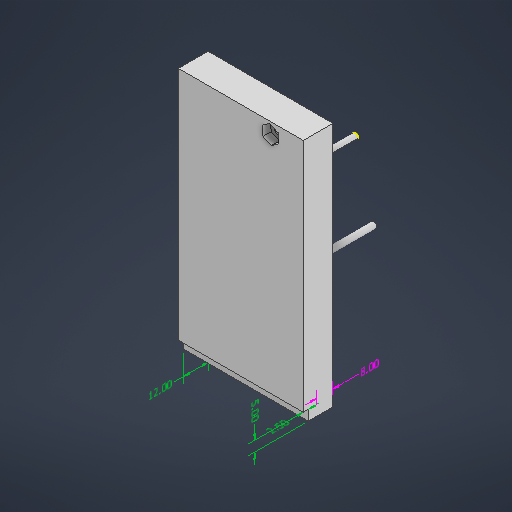
# Autodesk Inventor part: Cover of DC Housing
Saved by Autodesk Inventor 2026.2 (Build 302298010, 298A)
## iProperties
Created: 2026-04-19
Part Number: Cover of DC Housing
Material: Generic
Document SubType Name: Modeling
Designer: lenovo
Density: 1 g/cm^3
Appearance: Default
Author: lenovo
## iProperties of the stored document Cover of DC Housing_3DPrint.ipt
Created: 2026-04-19
Part Number: Cover of DC Housing_3DPrint
Material: Generic
Document SubType Name: Modeling
Designer: lenovo
Density: 1 g/cm^3
Appearance: Default
Author: lenovo
Autodesk Inventor part; units mm, degrees
ref_plane "YZ Plane" through (0, 0, 0) normal (1, 0, 0) x (0, 1, 0)
ref_plane "XZ Plane" through (0, 0, 0) normal (0, 1, 0) x (-1, 0, 0)
ref_plane "XY Plane" through (0, 0, 0) normal (0, 0, 1) x (1, 0, 0)
sketch "Sketch1" plane through (0, 0, 0) normal (0, 0, 1) x (1, 0, 0)
  line L0 (0, 0) -> (0, 120)
  line L1 (0, 120) -> (61, 120)
  line L2 (61, 120) -> (61, 0)
  line L3 (61, 0) -> (0, 0)
  line L4 (0, 5) -> (61, 5)
  line L5 (0, 110) -> (61, 110)
  dimension "d0" = 120
  dimension "d1" = 61
  dimension "d14" = 10
  dimension "d15" = 5
  constraints: 12 end point, 4 perpendicular, 4 point on line, 1 horizontal, 1 vertical
  measures "d0" distance of L0.start L0.end
  measures "d1" distance of L0.end L1.end
  measures "d14" distance between parallel lines of L5 L1
  measures "d15" distance between parallel lines of L3 L4
extrude "Extrusion1" add sketch "Sketch1" along normal blind 14.5 contours L0 L5 L2 L4 | L0 L1 L2 L5
extrude "Extrusion2" cut sketch "Sketch1" along normal blind 11.5 contours L0 L5 L2 L4
extrude "Extrusion3" add sketch "Sketch1" along normal blind 12 contours L0 L4 L2 L3
sketch "Sketch2" plane through (61, 5, 14.5) normal (1, 0, 0) x (0, 0, -1)
  line L0 (14.5, 115) -> (0, 115) projected
  line L1 (14.5, 115) -> (0, 115)
  line L2 (0, 0) -> (0, 115) projected
  line L3 (0, 115) -> (0, 0)
  line L4 (0, 0) -> (14.5, 0)
  line L5 (14.5, 0) -> (14.5, 115)
  point P0 (14.5, -5)
  constraints: 8 end point, 2 collinear, 2 perpendicular
extrude "Extrusion4" add sketch "Sketch2" against normal blind 1.5
sketch "Sketch3" plane through (0, 5, 14.5) normal (-1, 0, 0) x (0, 0, 1)
  line L0 (-14.5, 115) -> (-14.5, 105) projected
  line L1 (-14.5, 115) -> (0, 115) projected
  line L2 (-14.5, 115) -> (0, 115)
  line L3 (0, 0) -> (0, 115) projected
  line L4 (0, 115) -> (0, 0)
  line L5 (0, 0) -> (-14.5, 0)
  line L6 (-14.5, 0) -> (-14.5, 115)
  point P0 (-14.5, -5)
  constraints: 8 end point, 3 perpendicular, 1 horizontal
extrude "Extrusion5" add sketch "Sketch3" against normal blind 1.5
sketch "Sketch4" plane through (0, 0, 14.5) normal (0, 0, 1) x (1, 0, 0)
  circle A0 centre (45, 114.5) radius 2.25
  line L0 (61, 120) -> (0, 120) projected
  line L1 (45, 116.75) -> (46.9486, 115.625)
  line L2 (46.9486, 115.625) -> (46.9486, 113.375)
  line L3 (46.9486, 113.375) -> (45, 112.25)
  line L4 (45, 112.25) -> (43.0514, 113.375)
  line L5 (43.0514, 113.375) -> (43.0514, 115.625)
  line L6 (43.0514, 115.625) -> (45, 116.75)
  line L7 (0, 120) -> (0, 5) projected
  point P0 (0, 0)
  point P1 (30.5, 120)
  dimension "d23" = 4.5
  dimension "d60" = 45
  constraints: 12 end point, 1 coincident, 1 midpoint, 1 vertical alignment, 15 other
  measures "d60" distance from line of L7 point (45, 114.5)
hole "Hole1" at (45, 114.5, 14.5) direction (0, 0, -1) diameter 4.5 end through all counterbore diameter 9 counterbore depth 4
sketch "Sketch8" plane through (0, 0, 11.5) normal (0, 0, -1) x (-1, 0, 0)
  line L0 (-59.5, 110) -> (-1.5, 110) projected
  line L1 (-45, 110) -> (-45, 93)
  circle A0 centre (-45, 93) radius 1.4
  line L2 (-46.4, 93) -> (-43.6, 93)
  circle A1 centre (-36, 60) radius 1.4
  circle A2 centre (-54, 60) radius 1.4
  line L3 (-61, 0) -> (-61, 120) projected
  line L4 (-59.5, 110) -> (-59.5, 5) projected
  point P0 (0, 0)
  dimension "d45" = 17
  dimension "d46" = 2.8
  dimension "d56" = 2.8
  dimension "d57" = 2.8
  dimension "d66" = 33
  dimension "d67" = 33
  dimension "d68" = 9
  dimension "d69" = 18
  constraints: 4 end point, 3 centre point, 2 point on circle, 1 coincident, 1 vertical
  measures "d45" distance of L1.start L1.end
  measures "d46" diameter of A0
  measures "d56" diameter of A1
  measures "d57" diameter of A2
  measures "d66" vertical distance of A1.centre A0.centre
  measures "d67" vertical distance of A0.centre A2.centre
  measures "d68" horizontal distance of A1.centre A0.centre
  measures "d69" distance of A1.centre A2.centre
extrude "Extrusion8" add sketch "Sketch8" along normal blind 38.5 contours A0 L2 L1 | L1 L2 A0
sketch "Sketch9" plane through (0, 0, 14.5) normal (0, 0, 1) x (1, 0, 0)
  circle A0 centre (45, 114.5) radius 2.25 projected
  circle A1 centre (45, 114.5) radius 4.5 projected
  line L0 (48.665, 117.1111) -> (49.0938, 112.6316)
  line L1 (49.0938, 112.6316) -> (45.4288, 110.0205)
  line L2 (45.4288, 110.0205) -> (41.335, 111.8889)
  line L3 (41.335, 111.8889) -> (40.9062, 116.3684)
  line L4 (40.9062, 116.3684) -> (44.5712, 118.9795)
  line L5 (44.5712, 118.9795) -> (48.665, 117.1111)
  point P0 (0, 0)
  point P1 (45, 110)
  point P2 (44.5712, 118.9795)
  point P3 (44.5712, 118.9795)
  point P4 (40.9062, 116.3684)
  point P5 (40.9062, 116.3684)
  point P6 (41.335, 111.8889)
  point P7 (41.335, 111.8889)
  point P8 (49.0938, 112.6316)
  point P9 (45.4288, 110.0205)
  point P10 (49.0938, 112.6316)
  point P11 (45.4288, 110.0205)
  dimension "d53" = 8
  constraints: 12 end point, 1 coincident, 1 point on circle, 13 other
  measures "d53" distance of A1.end L0.start
extrude "Extrusion9" add sketch "Sketch9" against normal blind 4 contours A1 L0 | L5 A1 | L4 A1 | A1 L2 | L3 A1
extrude "Extrusion10" add sketch "Sketch9" against normal blind 4 contours A1 L1
sketch "Sketch10" plane through (45, 93, -27) normal (0, 0, -1) x (1, 0, 0)
  arc A0 (-1.4, 0) -> (1.4, 0) centre (0, 0) ccw projected
  line L0 (-1.4, 0) -> (1.4, 0)
  point P0 (-45, 93)
  constraints: 2 end point, 2 point on circle, 1 horizontal
extrude "Extrusion11" add sketch "Sketch8" along normal blind 38.5 contours A2
sketch "Sketch11" plane through (1.5, 5, 14.5) normal (1, 0, 0) x (0, 0, -1)
  line L0 (3, 105) -> (14.5, 105) projected
  line L1 (3, 105) -> (3, 56.18)
  line L2 (3, 0) -> (3, 105) projected
  line L3 (3, 56.18) -> (14.5, 56.18)
  line L4 (14.5, 115) -> (14.5, -5) projected
  line L5 (14.5, 56.18) -> (14.5, 54.18)
  line L6 (14.5, 54.18) -> (3, 54.18)
  line L7 (3, 54.18) -> (3, 56.18)
  point P0 (3, 54.18)
  dimension "d70" = 48.82
  dimension "d71" = 2
  constraints: 10 end point, 4 point on line, 3 perpendicular
  measures "d70" distance of L0.start L1.end
  measures "d71" distance of L3.end L5.end
extrude "Extrusion12" add sketch "Sketch11" along normal blind 47 contours L3 L4 L6 L2
body "Solid1"
